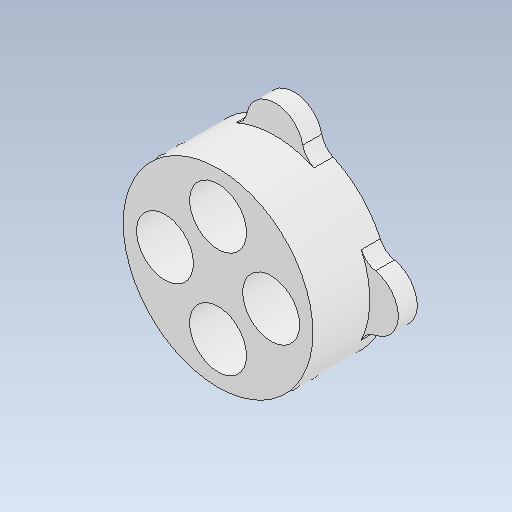
# Autodesk Inventor part: カムL4F
Saved by Autodesk Inventor 2020.2 (Build 242310000, 310)
## iProperties
Created: 2020-04-13
Part Number: カムL4F
Material: アセタール樹脂、白
Document SubType Name: Modeling
Designer: aoyama
Density: 1.425 g/cm^3
Appearance: 滑らか - 白
Author: aoyama
Autodesk Inventor part; units mm, degrees
ref_plane "YZ Plane" through (0, 0, 0) normal (1, 0, 0) x (0, 1, 0)
ref_plane "XZ Plane" through (0, 0, 0) normal (0, 1, 0) x (-1, 0, 0)
ref_plane "XY Plane" through (0, 0, 0) normal (0, 0, 1) x (1, 0, 0)
sketch "スケッチ1" plane through (0, 0, 0) normal (0, 0, 1) x (1, 0, 0)
  circle A0 centre (2.8, 0) radius 2.8
  line L0 (2.8, 0) -> (0, 0)
  circle A1 centre (0, 2.8) radius 2.8
  circle A2 centre (-2.8, 0) radius 2.8
  circle A3 centre (0, -2.8) radius 2.8
  circle A4 centre (2.8, 0) radius 1.5
  circle A5 centre (0, 2.8) radius 1.5
  circle A6 centre (-2.8, 0) radius 1.5
  circle A7 centre (0, -2.8) radius 1.5
  circle A8 centre (0, 0) radius 5
  circle A9 centre (0, 5) radius 1.5
  circle A10 centre (-5, 0) radius 1.5
  circle A11 centre (0, -5) radius 1.5
  circle A12 centre (5, 0) radius 1.5
  point P0 (-1.483, -4.775)
  point P1 (1.483, -4.775)
  point P2 (-4.775, -1.483)
  point P3 (-4.775, 1.483)
  point P4 (4.775, 1.483)
  point P5 (4.775, -1.483)
  point P6 (-1.483, 4.775)
  point P7 (1.483, 4.775)
  dimension "d12" = 10
  dimension "d1" = 5.6
  dimension "d4" = 360
  dimension "d7" = 3
  dimension "d10" = 360
  dimension "d15" = 3
  dimension "d18" = 360
  constraints: 12 centre point, 4 coincident, 2 end point, 1 equal radius, 1 horizontal, 32 other
  measures "d1" diameter of A0
  measures "d7" diameter of A4
  measures "d15" diameter of A9
extrude "押し出し1" add sketch "スケッチ1" along normal blind 4 contours A8 A12 A4 A1 A0 | A0 A1 A8 | A8 A12 A4 | A8 A3 A0 | A0 A3 A4 A12 A8 | A1 A4 A0 A5 | A0 A5 A9 A8 A1 | A3 A8 A11 A7 A0 | A0 A7 A3 A4 | A9 A5 A8 | A8 A11 A7 | A0 A2 A5 | A4 L0 A1 | A9 A5 A2 A1 A8 | A7 A2 A0 | A3 L0 A4 | A8 A3 A2 A7 A11 | A3 A6 A1 | A1 A6 A2 A5 | A2 A7 A3 A6 | A1 A2 A8 | A8 A2 A3 | A1 A6 A10 A8 A2 | A2 A8 A10 A6 A3 | A10 A6 A8
extrude "押し出し2" add sketch "スケッチ1" along normal blind 1 contours A0 A12 A8 | A0 A12 | A9 A8 A1 | A1 A9 | A11 A3 | A3 A11 A8 | A10 A8 A2 | A2 A10 picked at (5.3837, -0.1736) picked at (-0.1045, 5.1773) picked at (-0.1045, -5.1773) picked at (-5.1773, 0.1045)
fillet "フィレット1" radius 1.05 8 edges at (4.775, 1.483, 0.5) (4.775, -1.483, 0.5) (1.483, 4.775, 0.5) (-1.483, 4.775, 0.5) (-1.483, -4.775, 0.5) (1.483, -4.775, 0.5) (-4.775, 1.483, 0.5) (-4.775, -1.483, 0.5)
